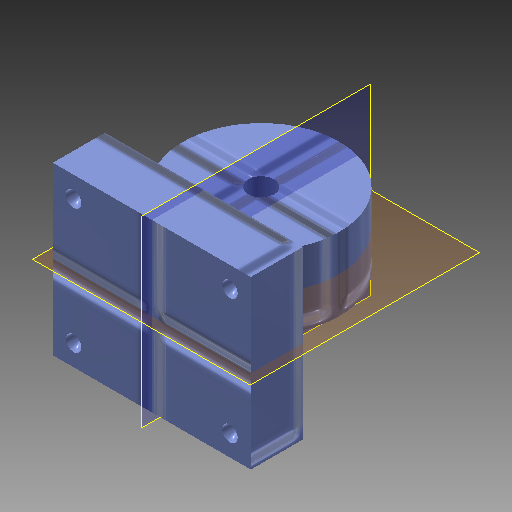
# Autodesk Inventor part: Roda-boba
Saved by Autodesk Inventor 2018 (Build 220112000, 112)
## iProperties
Created: 2016-05-10
Part Number: Roda-boba
Material: Genérico
Document SubType Name: Modeling
Designer: MarceloAdmin
Density: 1 g/cm^3
Appearance: Quadrado 4 pol - Azul claro
Author: MarceloAdmin
Autodesk Inventor part; units mm, degrees
ref_plane "YZ Plane" through (0, 0, 0) normal (1, 0, 0) x (0, 1, 0)
ref_plane "XZ Plane" through (0, 0, 0) normal (0, 1, 0) x (-1, 0, 0)
sketch "Esboço1" plane through (0, 0, 0) normal (0, 1, 0) x (-1, 0, 0)
  circle A0 centre (0, 0) radius 2.5
  circle A1 centre (0, 0) radius 15
  dimension "d0" = 5
  dimension "d1" = 30
  constraints: 2 centre point, 2 coincident
  measures "d0" diameter of A0
  measures "d1" diameter of A1
extrude "Extrusão1" add sketch "Esboço1" along normal blind 14
ref_plane "Plano de trabalho1" through (0, 0, 15) normal (0, 0, 1) x (1, 0, 0)
sketch "Esboço2" plane through (0, 0, 15) normal (0, 0, 1) x (1, 0, 0)
  line L0 (15, 14) -> (-15, 14) projected
  line L1 (-15, 0) -> (15, 0) projected
  line L2 (-15, 0) -> (-15, 14) projected
  line L3 (15, 0) -> (15, 14) projected
  line L4 (-15, 23) -> (23, 23)
  line L5 (23, 23) -> (23, -9)
  line L6 (23, -9) -> (-15, -9)
  line L7 (-15, -9) -> (-15, 23)
  point P0 (0, 0)
  point P1 (15, 7)
  dimension "d5" = 38
  dimension "d6" = 32
  dimension "d7" = 16
  dimension "d10" = 14
  constraints: 8 end point, 2 parallel, 1 horizontal, 1 midpoint, 1 perpendicular, 1 point on line
  measures "d5" distance between parallel lines of L5 L7
  measures "d6" distance between parallel lines of L4 L6
  measures "d7" distance from line of L4 point (15, 7)
  measures "d10" distance between parallel lines of L1 L0
extrude "Extrusão2" add sketch "Esboço2" along normal blind 10
sketch "Esboço3" plane through (0, 0, 25) normal (0, 0, 1) x (1, 0, 0)
  circle A0 centre (19, -5) radius 1.5
  circle A1 centre (-11, -5) radius 1.5
  circle A2 centre (-11, 19) radius 1.5
  circle A3 centre (19, 19) radius 1.5
  line L0 (23, -9) -> (23, 23) projected
  line L1 (23, 23) -> (-15, 23) projected
  line L2 (-15, -9) -> (23, -9) projected
  point P0 (0, 0)
  dimension "d11" = 3
  dimension "d12" = 3
  dimension "d13" = 3
  dimension "d14" = 3
  dimension "d15" = 24
  dimension "d16" = 24
  dimension "d17" = 30
  dimension "d18" = 30
  dimension "d19" = 30
  dimension "d20" = 24
  dimension "d21" = 32
  dimension "d22" = 4
  dimension "d23" = 38
  dimension "d24" = 4
  constraints: 4 centre point
  measures "d11" diameter of A0
  measures "d12" diameter of A1
  measures "d13" diameter of A2
  measures "d14" diameter of A3
  measures "d15" distance of A0.centre A3.centre
  measures "d16" distance of A1.centre A2.centre
  measures "d17" distance of A1.centre A0.centre
  measures "d18" distance of A2.centre A3.centre
  measures "d19" horizontal distance of A0.centre A2.centre
  measures "d20" vertical distance of A1.centre A3.centre
  measures "d21" distance of L0.start L0.end
  measures "d22" distance from line of L1 A3.centre
  measures "d23" distance of L2.start L0.start
  measures "d24" distance from line of L0 A0.centre
extrude "Extrusão3" cut sketch "Esboço3" against normal blind 10
ref_plane "Plano de trabalho2" through (4, -9, 15) normal (-1, 0, 0) x (0, 0, 1)
ref_plane "Plano de trabalho3" through (-15, 7, 15) normal (0, 1, 0) x (1, 0, 0)
equation "\"d16\" = d15"
equation "\"d22\" = -0.5 * d20 + 0.5 * d21"
equation "\"d24\" = -0.5 * d19 + 0.5 * d23"
